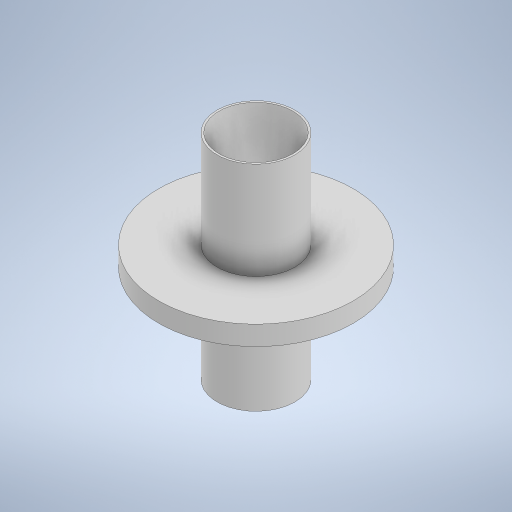
# Autodesk Inventor part: adapter
Saved by Autodesk Inventor 2023.1 (Build 271208000, 208)
## iProperties
Created: 2023-05-02
Part Number: adapter
Material: Generic
Document SubType Name: Modeling
Designer: dinesh
Density: 1 g/cm^3
Appearance: Default
Author: dinesh
Autodesk Inventor part; units mm, degrees
ref_plane "YZ Plane" through (0, 0, 0) normal (1, 0, 0) x (0, 1, 0)
ref_plane "XZ Plane" through (0, 0, 0) normal (0, 1, 0) x (-1, 0, 0)
ref_plane "XY Plane" through (0, 0, 0) normal (0, 0, 1) x (1, 0, 0)
sketch "Sketch1" plane through (0, 0, 0) normal (0, 0, 1) x (1, 0, 0)
  line L0 (0, 7.4625) -> (0, -7.4625)
  line L1 (-17.6657, 0) -> (17.6657, 0) construction
  line L2 (1, 0.5) -> (5, 0.5)
  line L3 (5, 0.5) -> (5, 0)
  line L4 (5, 0) -> (1, 0)
  line L5 (1, 0) -> (1, 0.5)
  line L6 (2, 0.5) -> (2, 5.5)
  line L7 (2, 5.5) -> (1.9, 5.5)
  line L8 (1.9, 5.5) -> (1, 0.5)
  line L9 (1, -0.5) -> (5, -0.5)
  line L10 (5, -0.5) -> (5, 0)
  line L11 (1, 0) -> (1, -0.5)
  line L12 (2, -0.5) -> (2, -5.5)
  line L13 (2, -5.5) -> (1.9, -5.5)
  line L14 (1.9, -5.5) -> (1, -0.5)
  point P0 (0, 0)
  point P1 (0, 0)
  dimension "d5" = 5
  dimension "d6" = 0.5
  dimension "d7" = 0.1
  dimension "d8" = 4
  dimension "d9" = 1
  dimension "d10" = 10
  constraints: 30 end point, 5 symmetric about line, 3 perpendicular, 3 point on line, 2 horizontal, 2 midpoint, 2 parallel, 1 coincident, 1 vertical
  measures "d5" distance of L6.start L6.end
  measures "d6" distance between parallel lines of L1 L2
  measures "d7" distance of L6.end L7.end
  measures "d8" diameter of L6 L0
  measures "d9" distance of L2.start L6.start
  measures "d10" diameter of L3 L0
revolve "Revolution1" add sketch "Sketch1" angle 360 about axis through (0, 7.4625, 0) along (0, -1, 0)
equation "\"d5\" = cn_h"
equation "\"d6\" = 0.5 * w_th"
equation "\"d7\" = tol"
equation "\"d8\" = t_D"
equation "\"d9\" = w_th"
equation "\"d10\" = top_D"
equation "\"tol\" = 0.1"
equation "\"w_th\" = 1"
equation "\"t_D\" = 4"
equation "\"top_D\" = 10"
equation "\"cn_h\" = 5"
equation "\"fillet_D\" = 2"
equation "\"w_l\" = 6"
equation "\"t_D_f\" = t_D + w_th"
equation "\"top_th\" = t_D + w_th"
equation "\"lv_OD\" = 26"
equation "\"lv_th\" = 1.5"
equation "\"sv_OD\" = 13"
equation "\"sv_th\" = 1.5"
equation "\"b_OD\" = 43.5"
equation "\"b_th\" = 1.5"
equation "\"b_ID\" = 37"
equation "\"b_rim_h\" = 5"
body "Solid1"
